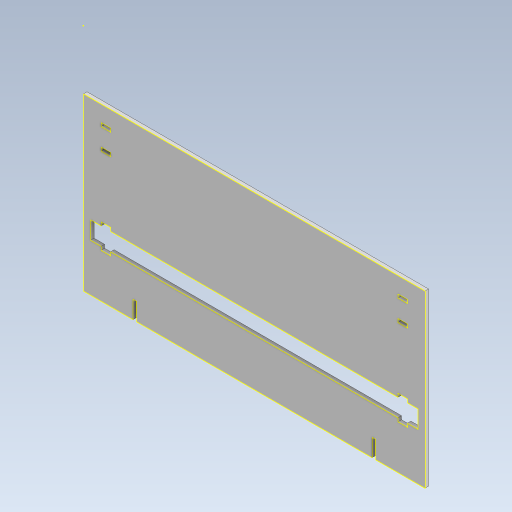
# Autodesk Inventor part: 零件5
Saved by Autodesk Inventor 2023 (Build 270158000, 158)
## iProperties
Created: 2023-05-12
Part Number: 零件5
Material: 一般
Document SubType Name: Modeling
Designer: Johnny Jou
Density: 1 g/cm^3
Appearance: 預設
Author: Johnny Jou
Autodesk Inventor part; units mm, degrees
ref_plane "YZ Plane" through (0, 0, 0) normal (1, 0, 0) x (0, 1, 0)
ref_plane "XZ Plane" through (0, 0, 0) normal (0, 1, 0) x (-1, 0, 0)
ref_plane "XY Plane" through (0, 0, 0) normal (0, 0, 1) x (1, 0, 0)
sketch "草圖1" plane through (0, 0, 0) normal (0, 0, 1) x (1, 0, 0)
  line L0 (0, 0) -> (290, 0)
  line L1 (290, 0) -> (290, -195)
  line L2 (290, -195) -> (0, -195)
  line L3 (0, -195) -> (0, 0)
  line L4 (15, -63.65) -> (23, -63.65)
  line L5 (23, -63.65) -> (23, -66.6)
  line L6 (23, -66.6) -> (15, -66.6)
  line L7 (15, -66.6) -> (15, -63.65)
  line L8 (15, -81.65) -> (23, -81.65)
  line L9 (23, -81.65) -> (23, -84.6)
  line L10 (23, -84.6) -> (15, -84.6)
  line L11 (15, -84.6) -> (15, -81.65)
  line L12 (15, -136.65) -> (23, -136.65)
  line L13 (23, -136.65) -> (23, -139.6)
  line L14 (23, -139.6) -> (15, -139.6)
  line L15 (15, -139.6) -> (15, -136.65)
  line L16 (15, -154.65) -> (23, -154.65)
  line L17 (23, -154.65) -> (23, -157.6)
  line L18 (23, -157.6) -> (15, -157.6)
  line L19 (15, -157.6) -> (15, -154.65)
  line L20 (275, -81.65) -> (275, -84.6)
  line L21 (275, -63.65) -> (275, -66.6)
  line L22 (267, -81.65) -> (275, -81.65)
  line L23 (275, -66.6) -> (267, -66.6)
  line L24 (267, -63.65) -> (275, -63.65)
  line L25 (275, -84.6) -> (267, -84.6)
  line L26 (267, -84.6) -> (267, -81.65)
  line L27 (267, -66.6) -> (267, -63.65)
  line L28 (267, -136.65) -> (275, -136.65)
  line L29 (275, -136.65) -> (275, -139.6)
  line L30 (267, -139.6) -> (267, -136.65)
  line L31 (275, -139.6) -> (267, -139.6)
  line L32 (267, -154.65) -> (275, -154.65)
  line L33 (275, -154.65) -> (275, -157.6)
  line L34 (275, -157.6) -> (267, -157.6)
  line L35 (267, -157.6) -> (267, -154.65)
  line L36 (0, -97.5) -> (290, -97.5) construction
  line L37 (19, -84.6) -> (19, -136.65) construction
  line L38 (145, 0) -> (145, -195) construction
  line L39 (23, -83.125) -> (267, -83.125) construction
  point P0 (15, -83.125)
  point P1 (15, -65.125)
  point P2 (15, -138.125)
  point P3 (15, -156.125)
  point P4 (267, -65.125)
  point P5 (267, -138.125)
  point P6 (267, -156.125)
  point P7 (145, -83.125)
  dimension "d0" = 2.95
  dimension "d1" = 8
  dimension "d2" = 18
  dimension "d3" = 55
  dimension "d4" = 18
  dimension "d5" = 195
  dimension "d6" = 290
  dimension "d9" = 252
  dimension "d16" = 12.9
  constraints: 80 end point, 12 midpoint, 11 point on line, 10 parallel, 6 horizontal, 6 perpendicular, 4 equal length, 36 other
  measures "d0" distance of L4.end L5.end
  measures "d1" distance of L4.start L4.end
  measures "d2" distance of point (15, -83.125) point (15, -65.125)
  measures "d3" distance of point (15, -138.125) point (15, -83.125)
  measures "d4" distance of point (15, -156.125) point (15, -138.125)
  measures "d5" distance of L0.end L1.end
  measures "d6" distance of L0.start L0.end
  measures "d9" distance of L5.end L21.end
  measures "d16" distance between parallel lines of L36 L10
extrude "擠出1" add sketch "草圖1" along normal blind 3
sketch "草圖3" plane through (0, 0, 3) normal (0, 0, 1) x (1, 0, 0)
  line L0 (290, 0) -> (0, 0) projected
  line L1 (0, 0) -> (290, 0)
  line L2 (290, 0) -> (290, -50)
  line L3 (290, -50) -> (0, -50)
  line L4 (0, -50) -> (0, 0)
  line L5 (290, -195) -> (290, 0) projected
  line L6 (42.05, -195) -> (45, -195)
  line L7 (45, -195) -> (45, -180)
  line L8 (45, -180) -> (42.05, -180)
  line L9 (42.05, -180) -> (42.05, -195)
  line L10 (0, -195) -> (290, -195) projected
  line L11 (245, -195) -> (247.95, -195)
  line L12 (247.95, -195) -> (247.95, -180)
  line L13 (247.95, -180) -> (245, -180)
  line L14 (245, -180) -> (245, -195)
  line L15 (45, -187.5) -> (245, -187.5)
  point P0 (145, -195)
  point P1 (145, -187.5)
  point P2 (247.95, -195)
  dimension "d17" = 50
  dimension "d18" = 200
  dimension "d19" = 2.95
  dimension "d20" = 2.95
  dimension "d22" = 15
  dimension "d23" = 0
  constraints: 26 end point, 6 parallel, 4 midpoint, 3 collinear, 3 horizontal, 3 perpendicular, 1 point on line
  measures "d17" distance of L1.end L2.end
  measures "d18" distance between parallel lines of L14 L7
  measures "d19" distance of L7.end L8.end
  measures "d20" distance of L12.end L13.end
  measures "d22" distance of L11.end L12.end
  measures "d23" horizontal distance of point (145, -195) point (145, -187.5)
extrude "擠出2" cut sketch "草圖3" against normal up to surface (3 mm away) contours L2 L3 L4 L0 | L9 L8 L7 L6 | L14 L13 L12 L10
sketch "草圖6" plane through (0, 0, 3) normal (0, 0, 1) x (1, 0, 0)
  line L0 (290, -66.6) -> (290, -81.65) projected
  line L1 (6, -139.6) -> (284, -139.6)
  line L2 (284, -139.6) -> (284, -154.65)
  line L3 (284, -154.65) -> (6, -154.65)
  line L4 (6, -154.65) -> (6, -139.6)
  line L5 (23, -139.6) -> (15, -139.6) projected
  line L6 (15, -154.65) -> (23, -154.65) projected
  line L7 (0, -50) -> (0, -195) projected
  line L8 (290, -195) -> (290, -50) projected
  point P0 (0, 0)
  point P1 (284, -147.125)
  dimension "d32" = 6
  dimension "d33" = 6
  constraints: 8 end point, 2 collinear, 2 parallel, 1 horizontal, 1 midpoint, 1 perpendicular
  measures "d32" distance between parallel lines of L7 L4
  measures "d33" distance from line of L8 point (284, -147.125)
extrude "擠出5" cut sketch "草圖6" against normal up to surface (3 mm away)
sketch "草圖7" plane through (0, 0, 3) normal (0, 0, 1) x (1, 0, 0)
  line L0 (15, -63.65) -> (23, -63.65) projected
  line L1 (23, -63.65) -> (23, -66.6) projected
  line L2 (23, -66.6) -> (15, -66.6) projected
  line L3 (15, -66.6) -> (15, -63.65) projected
  line L4 (15, -81.65) -> (23, -81.65) projected
  line L5 (23, -81.65) -> (23, -84.6) projected
  line L6 (23, -84.6) -> (15, -84.6) projected
  line L7 (15, -84.6) -> (15, -81.65) projected
  line L8 (275, -81.65) -> (275, -84.6) projected
  line L9 (275, -84.6) -> (267, -84.6) projected
  line L10 (267, -84.6) -> (267, -81.65) projected
  line L11 (267, -81.65) -> (275, -81.65) projected
  line L12 (275, -63.65) -> (275, -66.6) projected
  line L13 (275, -66.6) -> (267, -66.6) projected
  line L14 (267, -66.6) -> (267, -63.65) projected
  line L15 (267, -63.65) -> (275, -63.65) projected
  line L16 (15, -154.65) -> (6, -154.65) projected
  line L17 (6, -154.65) -> (6, -139.6) projected
  line L18 (6, -139.6) -> (15, -139.6) projected
  line L19 (15, -139.6) -> (15, -136.65) projected
  line L20 (15, -136.65) -> (23, -136.65) projected
  line L21 (23, -136.65) -> (23, -139.6) projected
  line L22 (23, -139.6) -> (267, -139.6) projected
  line L23 (267, -139.6) -> (267, -136.65) projected
  line L24 (267, -136.65) -> (275, -136.65) projected
  line L25 (275, -136.65) -> (275, -139.6) projected
  line L26 (275, -139.6) -> (284, -139.6) projected
  line L27 (284, -139.6) -> (284, -154.65) projected
  line L28 (284, -154.65) -> (275, -154.65) projected
  line L29 (275, -154.65) -> (275, -157.6) projected
  line L30 (275, -157.6) -> (267, -157.6) projected
  line L31 (267, -157.6) -> (267, -154.65) projected
  line L32 (267, -154.65) -> (23, -154.65) projected
  line L33 (23, -154.65) -> (23, -157.6) projected
  line L34 (23, -157.6) -> (15, -157.6) projected
  line L35 (15, -157.6) -> (15, -154.65) projected
  line L36 (247.95, -180) -> (247.95, -195) projected
  line L37 (247.95, -195) -> (290, -195) projected
  line L38 (290, -195) -> (290, -50) projected
  line L39 (290, -50) -> (0, -50) projected
  line L40 (0, -50) -> (0, -195) projected
  line L41 (0, -195) -> (42.05, -195) projected
  line L42 (42.05, -195) -> (42.05, -180) projected
  line L43 (42.05, -180) -> (45, -180) projected
  line L44 (45, -180) -> (45, -195) projected
  line L45 (45, -195) -> (245, -195) projected
  line L46 (245, -195) -> (245, -180) projected
  line L47 (245, -180) -> (247.95, -180) projected
  point P0 (0, 0)
